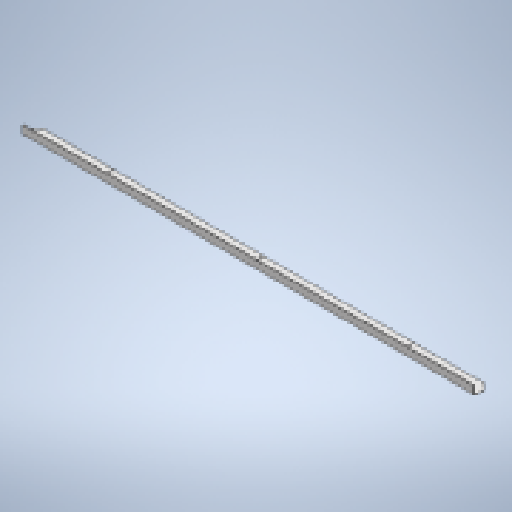
# Autodesk Inventor part: МОО 051 стрингер спина 1
Saved by Autodesk Inventor 2024.2 (Build 282272000, 272)
## iProperties
Created: 2024-04-28
Part Number: МОО 051 стрингер спина 1
Material: Stainless Steel
Document SubType Name: Sheet Metal
Designer: pokla
Density: 8 g/cm^3
Sheet Metal Rule: AISI304 2mm Die16
Appearance: Default
Flat Pattern Width: 7.79478 cm
Flat Pattern Length: 150 cm
Flat Pattern Area: 1169.22 cm^2
Sheet Metal Width: 77,948 mm
Sheet Metal Length: 1500,000 mm
Sheet Metal Area: 116921,741 mm^2
Author: admin
Autodesk Inventor part; units mm, degrees
ref_plane "YZ Plane" through (0, 0, 0) normal (1, 0, 0) x (0, 1, 0)
ref_plane "XZ Plane" through (0, 0, 0) normal (0, 1, 0) x (-1, 0, 0)
ref_plane "XY Plane" through (0, 0, 0) normal (0, 0, 1) x (1, 0, 0)
sketch "Sketch1" plane through (0, 0, 0) normal (0, 0, 1) x (1, 0, 0)
  line L0 (-750, 51.7458) -> (750, 51.7458)
  line L1 (750, 51.7458) -> (750, 0)
  line L2 (750, 0) -> (-750, 0)
  line L3 (-750, 0) -> (-750, 51.7458)
  point P0 (0, 0)
  point P1 (0, 0)
  dimension "d0" = 1500
  dimension "d1" = 51.7458
  measures "d0" distance of L1.end L2.end
  measures "d1" distance of L0.end L1.end
extrude "Plate1" add sketch "Sketch1" along normal blind 2
sketch "Sketch2" plane through (750, 2, 0) normal (0, -1, 0) x (1, 0, 0)
  line L0 (-1500, 0) -> (0, 0)
  line L1 (0, 0) -> (0, 30)
  line L2 (0, 30) -> (-1500, 30)
  line L3 (-1500, 30) -> (-1500, 0)
  constraints: 6 end point, 1 horizontal, 1 perpendicular, 1 vertical
edge flange "Flange1" height 30 angle 90 thickness 2 bend radius 2.75 thickness toward (0, -1, 0) relief round relief width 2 relief depth 1 edges at (0, 0, 2) wall of the first edge with corners at (-750, 2, 0) (750, 2, 0) (750, 2, 30) (-750, 2, 30)
bend "Bend1"
corner "Corner1"
sketch "Sketch5" plane through (0, 0, 0) normal (0, 0, -1) x (-1, 0, 0)
  line L0 (750, 51.7458) -> (-750, 51.7458) projected
  line L1 (-1, 30) -> (-1, 51.7458)
  line L2 (750, 0) -> (-750, 0) projected
  line L3 (-1, 30) -> (1, 30)
  line L4 (1, 30) -> (1, 51.7458)
  point P0 (0, 0)
  point P1 (0, 30)
  point P2 (0, 0)
  dimension "d27" = 2
  dimension "d29" = 30
  constraints: 6 end point, 2 midpoint, 2 point on line, 1 horizontal, 1 parallel, 1 perpendicular, 1 vertical alignment
  measures "d27" distance of L1.start L3.end
  measures "d29" distance from line of L2 L3.end
extrude "Extrusion1" cut sketch "Sketch5" against normal through all
pattern_linear "Rectangular Pattern1" count 3 spacing 500 along (1, 0, 0) of "Extrusion1" first direction both ways yes
sketch "Sketch6" plane through (0, 0, 0) normal (0, 0, -1) x (-1, 0, 0)
  line L0 (-750, 51.7458) -> (-750, 4.75) projected
  circle A0 centre (-750, 51.7458) radius 15
  line L1 (-750, 51.7458) -> (750, 51.7458) projected
  point P0 (0, 0)
  point P1 (-502, 51.9458)
  point P2 (-735, 51.7458)
  point P3 (-750, 36.7458)
  point P4 (750, 51.7458)
  dimension "d24" = 30
  constraints: 1 centre point, 1 other
  measures "d24" diameter of A0
extrude "Extrusion2" cut sketch "Sketch6" against normal through all contours L1 A0 L0 picked at (-740.1254, 50.6332)
mirror "Mirror1" about plane through (0, 0, 0) normal (1, 0, 0) of "Extrusion2"
sketch "Sketch7" plane through (0, 0, 2) normal (0, 0, 1) x (1, 0, 0)
  arc A0 (-750, 36.7458) -> (-735, 51.7458) centre (-750, 51.7458) ccw projected
  line L0 (-750, 4.75) -> (-750, 36.7458) projected
  line L1 (-750, 4.75) -> (750, 4.75) projected
  line L2 (750, 36.7458) -> (750, 4.75) projected
  arc A1 (735, 51.7458) -> (750, 36.7458) centre (750, 51.7458) ccw projected
  line L3 (501, 51.7458) -> (735, 51.7458) projected
  line L4 (501, 51.7458) -> (501, 30) projected
  line L5 (501, 30) -> (499, 30) projected
  line L6 (499, 30) -> (499, 51.7458) projected
  line L7 (1, 51.7458) -> (499, 51.7458) projected
  line L8 (1, 51.7458) -> (1, 30) projected
  line L9 (1, 30) -> (-1, 30) projected
  line L10 (-1, 30) -> (-1, 51.7458) projected
  line L11 (-499, 51.7458) -> (-1, 51.7458) projected
  line L12 (-499, 51.7458) -> (-499, 30) projected
  line L13 (-499, 30) -> (-501, 30) projected
  line L14 (-501, 30) -> (-501, 51.7458) projected
  line L15 (-735, 51.7458) -> (-501, 51.7458) projected
  line L16 (649, 24.2479) -> (651, 24.2479)
  line L17 (651, 24.2479) -> (651, 32.2479)
  line L18 (651, 32.2479) -> (649, 32.2479)
  line L19 (649, 32.2479) -> (649, 24.2479)
  line L20 (650, 4.75) -> (650, 51.7458) construction
  point P0 (0, 0)
  point P1 (650, 24.2479)
  point P2 (649, 28.2479)
  point P3 (650, 28.2479)
  dimension "d30" = 2
  dimension "d31" = 8
  dimension "d33" = 100
  constraints: 10 end point, 3 midpoint, 2 parallel, 2 perpendicular, 2 point on line, 1 horizontal, 1 horizontal alignment, 1 vertical alignment
  measures "d30" distance of L18.end L17.end
  measures "d31" distance of L16.end L17.end
  measures "d33" distance between parallel lines of L20 L2
extrude "Extrusion3" cut sketch "Sketch7" along normal through all both and the other way through all contours L19 L18 L17 L16
mirror "Mirror2" about plane through (0, 0, 0) normal (1, 0, 0) of "Extrusion3"
sketch "Sketch8" plane through (0, 0, 0) normal (0, 0, -1) x (-1, 0, 0)
  line L0 (-472.8473, 35.5904) -> (-272.8473, 35.5904) construction
  line L1 (-272.8473, 35.5904) -> (-272.8473, 15.5904) construction
  line L2 (-272.8473, 15.5904) -> (-472.8473, 15.5904) construction
  line L3 (-472.8473, 15.5904) -> (-472.8473, 35.5904) construction
  point P0 (0, 0)
  dimension "d36" = 200
  dimension "d37" = 20
  constraints: 1 horizontal, 2 other
  measures "d36" distance of L3.end L0.end
  measures "d37" distance of L0.end L1.end
mark "Mark1"
equation "\"d1\" = Стрингер_1"
equation "\"d27\" = d18"
equation "\"d29\" = Стрингер_глубина_паза"
equation "\"d2\" = Thickness"
equation "\"d3\" = BendReliefWidth"
equation "\"d4\" = BendReliefDepth"
equation "\"d5\" = MinimumRemnant"
equation "\"d6\" = TransitionRadius"
equation "\"d9\" = BendRadius"
equation "\"d10\" = CornerReliefSize"
equation "\"d11\" = GapSize"
equation "\"d12\" = JacobiRadiusSize"
equation "\"GapSize\" = Thickness"
equation "\"MinimumRemnant\" = 2 * Thickness"
equation "\"BendReliefDepth\" = 0.5 * Thickness"
equation "\"BendReliefWidth\" = Thickness"
equation "\"CornerReliefSize\" = 4 * Thickness"
equation "\"JacobiRadiusSize\" = BendRadius"
equation "\"TransitionRadius\" = BendRadius"
equation "\"d18\" = Thickness"
equation "\"qqqqqq\" = 67.35706"
equation "\"Стрингер_1\" = 51.745837"
equation "\"Стрингер_глубина_паза\" = 30"
equation "\"Thickness\" = 2"
equation "\"BendRadius\" = 2.75"
body "Solid1"
